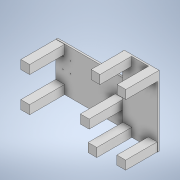
# Autodesk Inventor part: Estructura de soporte
Saved by Autodesk Inventor 2020 (Build 240168000, 168)
## iProperties
Created: 2020-11-30
Part Number: Estructura de soporte
Material: Generic
Document SubType Name: Modeling
Designer: Daniel
Density: 1 g/cm^3
Appearance: Default
Author: Daniel
Autodesk Inventor part; units mm, degrees
ref_plane "YZ Plane" through (0, 0, 0) normal (1, 0, 0) x (0, 1, 0)
ref_plane "XZ Plane" through (0, 0, 0) normal (0, 1, 0) x (-1, 0, 0)
ref_plane "XY Plane" through (0, 0, 0) normal (0, 0, 1) x (1, 0, 0)
sketch "Sketch1" plane through (0, 0, 0) normal (0, 0, 1) x (1, 0, 0)
  line L0 (0, 0) -> (1524, 0)
  line L1 (1524, 0) -> (1524, 1016)
  line L2 (1524, 1016) -> (1016, 1016)
  line L3 (1016, 1016) -> (1016, 635)
  line L4 (1016, 635) -> (0, 635)
  line L5 (0, 635) -> (0, 0)
  dimension "d0" = 1524
  dimension "d1" = 1016
  dimension "d2" = 508
  dimension "d3" = 381
  constraints: 12 end point, 3 perpendicular, 2 horizontal, 1 vertical
  measures "d0" distance of L0.start L0.end
  measures "d1" distance of L0.end L1.end
  measures "d2" distance of L1.end L2.end
  measures "d3" distance of L2.end L3.end
extrude "Extrusion1" add sketch "Sketch1" along normal blind 25.4
sketch "Sketch2" plane through (0, 0, 25.4) normal (0, 0, 1) x (1, 0, 0)
  line L0 (0, 631.4106) -> (127, 631.4106)
  line L1 (127, 631.4106) -> (127, 504.4106)
  line L2 (127, 504.4106) -> (0, 504.4106)
  line L3 (0, 504.4106) -> (0, 631.4106)
  line L4 (0, 635) -> (0, 0) projected
  line L5 (0, 0) -> (127, 0)
  line L6 (127, 0) -> (127, 127)
  line L7 (127, 127) -> (0, 127)
  line L8 (0, 127) -> (0, 0)
  line L9 (1520.8454, 0) -> (1393.8454, 0)
  line L10 (1393.8454, 0) -> (1393.8454, 127)
  line L11 (1393.8454, 127) -> (1520.8454, 127)
  line L12 (1520.8454, 127) -> (1520.8454, 0)
  line L13 (1524, 1016) -> (1016, 1016) projected
  line L14 (1524, 1016) -> (1397, 1016)
  line L15 (1397, 1016) -> (1397, 889)
  line L16 (1397, 889) -> (1524, 889)
  line L17 (1524, 889) -> (1524, 1016)
  line L18 (1020.6484, 1016) -> (1147.6484, 1016)
  line L19 (1147.6484, 1016) -> (1147.6484, 889)
  line L20 (1147.6484, 889) -> (1020.6484, 889)
  line L21 (1020.6484, 889) -> (1020.6484, 1016)
  dimension "d6" = 127
  dimension "d7" = 127
  dimension "d8" = 127
  dimension "d9" = 127
  dimension "d10" = 127
  dimension "d11" = 127
  dimension "d12" = 127
  dimension "d13" = 127
  dimension "d14" = 127
  dimension "d15" = 127
  constraints: 40 end point, 10 parallel, 5 horizontal, 5 perpendicular, 2 point on line
  measures "d6" distance of L1.end L2.end
  measures "d7" distance of L0.end L1.end
  measures "d8" distance of L7.end L6.end
  measures "d9" distance of L6.end L5.end
  measures "d10" distance of L10.end L11.end
  measures "d11" distance of L9.end L10.end
  measures "d12" distance of L16.end L15.end
  measures "d13" distance of L15.end L14.end
  measures "d14" distance of L19.end L20.end
  measures "d15" distance of L18.end L19.end
extrude "Extrusion2" add sketch "Sketch2" along normal blind 508
sketch "Sketch3" plane through (0, 0, 0) normal (0, 0, -1) x (-1, 0, 0)
  circle A0 centre (-101.6, 466.3106) radius 5.9944
  circle A1 centre (-101.6, 304.4618) radius 5.9944
  circle A2 centre (-211.6074, 304.4618) radius 5.9944
  circle A3 centre (-211.6074, 466.3106) radius 5.9944
  line L0 (-127, 504.4106) -> (0, 504.4106) projected
  line L1 (0, 635) -> (0, 0) projected
  dimension "d18" = 11.9888
  dimension "d19" = 11.9888
  dimension "d20" = 11.9888
  dimension "d21" = 11.9888
  dimension "d23" = 38.1
  dimension "d24" = 161.8488
  dimension "d25" = 110.0074
  dimension "d26" = 110.0074
  dimension "d27" = 101.6
  constraints: 4 centre point, 2 horizontal alignment, 1 vertical alignment
  measures "d18" diameter of A0
  measures "d19" diameter of A1
  measures "d20" diameter of A2
  measures "d21" diameter of A3
  measures "d23" distance from line of A0.centre L0
  measures "d24" distance of A1.centre A0.centre
  measures "d25" distance of A2.centre A1.centre
  measures "d26" distance of A3.centre A0.centre
  measures "d27" distance from line of A0.centre L1
extrude "Extrusion3" cut sketch "Sketch3" against normal blind 508
sketch "Sketch4" plane through (0, 0, 0) normal (0, 0, -1) x (-1, 0, 0)
  line L0 (-1016, 635) -> (0, 635) projected
  line L1 (-1016, 635) -> (-1016, 0)
  line L2 (-127, 0) -> (-1393.8454, 0) projected
  line L3 (0, 0) -> (-1524, 0) projected
  line L4 (-1016, 0) -> (-1524, 0)
  line L5 (-1524, 0) -> (-1524, 1016) projected
  line L6 (-1524, 0) -> (-1524, 1016)
  line L7 (-1524, 1016) -> (-1016, 1016)
  line L8 (-1016, 1016) -> (-1016, 635) projected
  line L9 (-1016, 1016) -> (-1016, 635)
  constraints: 10 end point, 2 perpendicular, 2 point on line, 1 collinear, 1 horizontal, 1 vertical
extrude "Extrusion4" add sketch "Sketch4" against normal blind 76.2
sketch "Sketch5" plane through (0, 0, 0) normal (0, 0, -1) x (-1, 0, 0)
  line L0 (-1524, 889) -> (-1524, 1016) projected
  line L1 (-1016, 0) -> (-1524, 0)
  line L2 (-1524, 0) -> (-1524, 1016)
  line L3 (-1524, 1016) -> (-1016, 1016)
  line L4 (-1016, 1016) -> (-1016, 0)
  point P0 (0, 0)
  constraints: 8 end point, 2 parallel, 1 horizontal, 1 perpendicular
extrude "Extrusion5" cut sketch "Sketch5" against normal blind 50.8
sketch "Sketch7" plane through (0, 0, 25.4) normal (0, 0, 1) x (1, 0, 0)
  line L0 (863.6, 377.9671) -> (990.6, 377.9671)
  line L1 (990.6, 377.9671) -> (990.6, 250.9671)
  line L2 (990.6, 250.9671) -> (863.6, 250.9671)
  line L3 (863.6, 250.9671) -> (863.6, 377.9671)
  line L4 (0, 504.4106) -> (0, 127) projected
  point P0 (0, 0)
  dimension "d40" = 127
  dimension "d41" = 127
  dimension "d42" = 863.6
  constraints: 8 end point, 2 parallel, 1 horizontal, 1 perpendicular
  measures "d40" distance of L1.end L2.end
  measures "d41" distance of L0.end L1.end
  measures "d42" distance between parallel lines of L4 L3
extrude "Extrusion6" add sketch "Sketch7" along normal blind 508
sketch "Sketch8" plane through (0, 0, 76.2) normal (0, 0, 1) x (1, 0, 0)
  line L0 (1025.8462, 0) -> (1152.8462, 0)
  line L1 (1152.8462, 0) -> (1152.8462, 127)
  line L2 (1152.8462, 127) -> (1025.8462, 127)
  line L3 (1025.8462, 127) -> (1025.8462, 0)
  point P0 (0, 0)
  dimension "d45" = 127
  dimension "d46" = 127
  constraints: 8 end point, 2 parallel, 1 horizontal, 1 perpendicular
  measures "d45" distance of L2.end L1.end
  measures "d46" distance of L1.end L0.end
extrude "Extrusion7" add sketch "Sketch8" along normal blind 508
body "Solid1"
